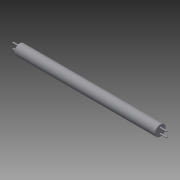
# Autodesk Inventor part: świetlówka
Saved by Autodesk Inventor 2014 (Build 180170000, 170)
## iProperties
Created: 2013-12-25
Part Number: świetlówka
Material: Ogólny
Document SubType Name: Modeling
Designer: Kuba
Density: 1 g/cm^3
Appearance: Domyślna
Author: Kuba
Autodesk Inventor part; units mm, degrees
ref_plane "YZ Plane" through (0, 0, 0) normal (1, 0, 0) x (0, 1, 0)
ref_plane "XZ Plane" through (0, 0, 0) normal (0, 1, 0) x (-1, 0, 0)
ref_plane "XY Plane" through (0, 0, 0) normal (0, 0, 1) x (1, 0, 0)
sketch "Szkic1" plane through (0, 0, 0) normal (1, 0, 0) x (0, 1, 0)
  line L0 (-11.2, 0) -> (11.2, 0) projected
  line L1 (0, -11.2) -> (0, 11.2) projected
  circle A0 centre (0, 0) radius 8
  dimension "d0" = 16
  constraints: 1 centre point, 1 coincident
  measures "d0" diameter of A0
extrude "Wyciągnięcie proste1" add sketch "Szkic1" along normal blind 212
sketch "Szkic2" plane through (212, 0, 0) normal (1, 0, 0) x (0, 0, -1)
  circle A0 centre (0, 0) radius 8 projected
  line L0 (0, -11.2) -> (0, 11.2) projected
  line L1 (16, 0) -> (-12, 0) projected
  circle A1 centre (-4, 0) radius 1
  circle A2 centre (4, 0) radius 1
  point P0 (12, 0)
  dimension "d4" = 16
  dimension "d5" = 2
  dimension "d8" = 8
  constraints: 2 centre point, 2 point on line, 1 coincident, 1 horizontal, 1 symmetric about line, 3 other
  measures "d4" diameter of A0
  measures "d5" diameter of A1
  measures "d8" distance of A1.centre A2.centre
extrude "Wyciągnięcie proste2" add sketch "Szkic2" along normal blind 7 contours A2 L1 | L1 A2 | A1 L1 | L1 A1
sketch "Szkic3" plane through (0, 0, 0) normal (-1, 0, 0) x (0, 0, 1)
  circle A0 centre (0, 0) radius 8 projected
  line L0 (-11.2, 0) -> (11.2, 0) projected
  line L1 (0, -11.2) -> (0, 11.2) projected
  circle A1 centre (-4, 0) radius 1
  circle A2 centre (4, 0) radius 1
  dimension "d19" = 10
  dimension "d15" = 2
  dimension "d16" = 16
  dimension "d22" = 8
  constraints: 2 centre point, 1 horizontal, 1 point on line, 1 symmetric about line, 2 other
  measures "d15" diameter of A1
  measures "d16" diameter of A0
  measures "d22" distance of A1.centre A2.centre
extrude "Wyciągnięcie proste3" add sketch "Szkic3" along normal blind 7 contours A2 L0 | L0 A2 | A1 L0 | L0 A1
equation "\"d8\" = 0.5 * d4"
equation "\"d22\" = 0.5 * d16"
